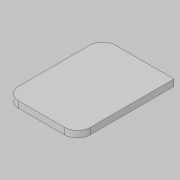
# Autodesk Inventor part: picaseV2lid
Saved by Autodesk Inventor 2018.3 (Build 223284000, 284)
## iProperties
Created: 2018-03-01
Part Number: picaseV2lid
Material: Generic
Document SubType Name: Modeling
Designer: mjsi2
Density: 1 g/cm^3
Appearance: Default
Author: mjsi2
Autodesk Inventor part; units mm, degrees
ref_plane "YZ Plane" through (0, 0, 0) normal (1, 0, 0) x (0, 1, 0)
ref_plane "XZ Plane" through (0, 0, 0) normal (0, 1, 0) x (-1, 0, 0)
ref_plane "XY Plane" through (0, 0, 0) normal (0, 0, 1) x (1, 0, 0)
sketch "Sketch1" plane through (0, 0, 0) normal (0, 1, 0) x (-1, 0, 0)
  line L0 (79.7789, 88.5449) -> (79.7789, -61.4551)
  line L1 (79.7789, -61.4551) -> (-31.0159, -61.4551)
  line L2 (-31.0159, -61.4551) -> (-31.0159, 88.5449)
  line L3 (-31.0159, 88.5449) -> (79.7789, 88.5449)
  point P0 (0, 0)
  dimension "d0" = 150
  dimension "d1" = 110.7948
  constraints: 8 end point, 1 parallel, 1 perpendicular
  measures "d0" distance of L0.start L0.end
  measures "d1" distance of L0.end L1.end
extrude "Body" add sketch "Sketch1" along normal blind 10
fillet "Fillet6" radius 20 1 edges at (-79.7789, 5, -61.4551)
fillet "Fillet4" radius 20 1 edges at (-79.7789, 5, 88.5449)
fillet "Fillet2" radius 20 1 edges at (31.0159, 5, 88.5449)
shell "Shell2" thickness 2 removed faces 1 at (-42.8473, 0, 31.8782)
body "Solid1"
